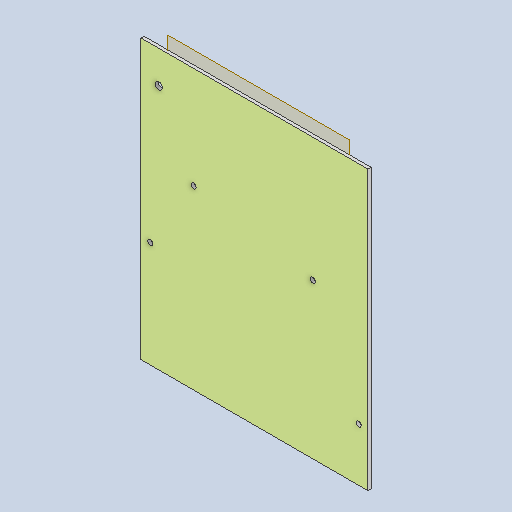
# Autodesk Inventor part: Z axis front plate
Saved by Autodesk Inventor 2023.2 (Build 272271000, 271)
## iProperties
Created: 2023-02-16
Part Number: Z axis front plate
Material: Generic
Document SubType Name: Modeling
Designer: dmargari
Density: 1 g/cm^3
Appearance: Default
Author: dmargari
Autodesk Inventor part; units mm, degrees
ref_plane "YZ Plane" through (0, 0, 0) normal (1, 0, 0) x (0, 1, 0)
ref_plane "XZ Plane" through (0, 0, 0) normal (0, 1, 0) x (-1, 0, 0)
ref_plane "XY Plane" through (0, 0, 0) normal (0, 0, 1) x (1, 0, 0)
ref_plane "Work Plane1" through (-9, 0, -3.2032) normal (0, 0, 1) x (1, 0, 0)
sketch "Sketch1" plane through (-9, 0, -3.2032) normal (0, 0, 1) x (1, 0, 0)
  ellipse E0 centre (-38.5, 0) end of major axis (-36.433, 0) minor radius 2.0669 projected
  ellipse E1 centre (36.5, 0) end of major axis (38.567, 0) minor radius 2.0669 projected
  line L0 (89, -44.9989) -> (89, 224.9989)
  line L1 (-111, 224.9989) -> (-111, -44.9989)
  line L2 (-111, -44.9989) -> (89, -44.9989)
  line L3 (89, 224.9989) -> (-91, 224.9989) projected
  line L4 (-91, -24.9989) -> (-91, 224.9989) projected
  line L5 (-91, -24.9989) -> (89, -24.9989) projected
  line L6 (89, 224.9989) -> (89, -24.9989) projected
  line L7 (-91, 224.9989) -> (-111, 224.9989)
  line L8 (89, -44.9989) -> (109, -44.9989)
  line L9 (109, -44.9989) -> (109, 224.9989)
  line L10 (109, 224.9989) -> (89, 224.9989)
  line L11 (89, 224.9989) -> (-91, 224.9989)
  point P0 (9, 0)
  point P1 (79, 224.9989)
  point P2 (79, -24.9989)
  point P3 (-81, 224.9989)
  point P4 (-81, -24.9989)
  point P5 (-91, 1846.3654)
  dimension "d40" = 20
  dimension "d41" = 90
  constraints: 16 end point, 2 perpendicular, 2 point on line, 1 collinear, 1 horizontal
  measures "d40" distance of L0.start L8.end
  measures "d41" angle of L9 L8
extrude "Extrusion1" add sketch "Sketch1" along normal blind 3 contours E0 | E1 | L2 L1 L7 L4 L5 L0 | L0 L10 L9 L8 | L5 L4 L3 L0
sketch "Sketch2" plane through (-9, 0, -0.2032) normal (0, 0, 1) x (1, 0, 0)
  line L0 (-111, -44.9989) -> (89, -44.9989) construction
  line L1 (55.5, -44.9989) -> (55.5, 235.0161) construction
  line L2 (89, -44.9989) -> (89, 224.9989) construction
  line L3 (88.5, -24.9989) -> (88.5, 475.0011) projected
  point P0 (9, 0)
  point P1 (89, 4927.5367)
  point P2 (55.5, 105.0011)
  dimension "d4" = 33
  dimension "d12" = 150
  constraints: 2 end point, 2 point on line, 1 vertical
  measures "d4" distance between parallel lines of L3 L1
  measures "d12" distance from line of L0 point (55.5, 105.001)
hole "Hole1" at (46.5, 105.0011, -0.2032) direction (0, 0, -1) diameter 5.1 depth 3
sketch "Sketch3" plane through (-9, 0, -0.2032) normal (0, 0, 1) x (1, 0, 0)
  line L0 (89, -24.9989) -> (89, -24.9989) projected
  line L1 (89, -24.9989) -> (89, 475.0011) projected
  line L2 (89, 475.0011) -> (89, 475.0011) projected
  line L3 (89, -24.9989) -> (89, 475.0011) projected
  line L4 (69, -24.9989) -> (69, -24.9989) projected
  line L5 (69, -24.9989) -> (69, 475.0011) projected
  line L6 (69, 475.0011) -> (69, 475.0011) projected
  line L7 (69, -24.9989) -> (69, 475.0011) projected
  line L8 (-91, -24.9989) -> (-91, -24.9989) projected
  line L9 (-91, -24.9989) -> (-91, 475.0011) projected
  line L10 (-91, 475.0011) -> (-91, 475.0011) projected
  line L11 (-91, -24.9989) -> (-91, 475.0011) projected
  line L12 (-71, -24.9989) -> (-71, -24.9989) projected
  line L13 (-71, -24.9989) -> (-71, 475.0011) projected
  line L14 (-71, 475.0011) -> (-71, 475.0011) projected
  line L15 (-71, -24.9989) -> (-71, 475.0011) projected
  line L16 (100, -24.9989) -> (100, 239.9989) construction
  line L17 (-102, -24.9989) -> (-102, 244.9989) construction
  line L18 (-60, -24.9989) -> (-60, 2205.8354) construction
  line L19 (98.966, 4926.9545) -> (-101.034, 1503.4308) construction
  line L20 (55.3, -24.9989) -> (55.3, 4179.4968) construction
  line L21 (89, -44.9989) -> (89, 224.9989) projected
  point P0 (9, 0)
  point P1 (89, 4927.5367)
  point P2 (-111, 1504.013)
  point P3 (100, 6.4871)
  point P4 (-60, 126.3923)
  point P5 (-102, 57.9278)
  point P6 (-102, 193.5737)
  dimension "d14" = 11
  dimension "d15" = 11
  dimension "d16" = 13.7
  dimension "d39" = 11
  constraints: 8 end point, 4 point on line, 4 vertical, 3 other
  measures "d14" distance between parallel lines of L11 L17
  measures "d15" distance between parallel lines of L18 L15
  measures "d16" distance between parallel lines of L7 L20
  measures "d39" distance between parallel lines of L3 L16
hole "Hole3" at (91, 6.4871, -0.2032) at (-69, 126.3923, -0.2032) at (-111, 57.9278, -0.2032) direction (0, 0, -1) diameter 5.1 depth 3
sketch "Sketch4" plane through (-9, 0, -0.2032) normal (0, 0, 1) x (1, 0, 0)
  point P0 (9, 0)
  point P1 (-93.7009, 193.5736)
hole "Hole4" at (-102.7009, 193.5736, -0.2032) direction (0, 0, -1) diameter 7.1 depth 3
